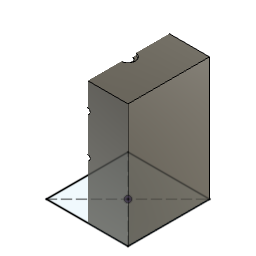
Ikea Stubby Leg v1 (Autodesk Fusion 360 design; units mm, degrees)
Autodesk Fusion 360 part; units mm, degrees
sketch "Sketch1" plane through (0, 0, 0) normal (0, 0, 1) x (1, 0, 0)
  line L0 (25.2, -25.2) -> (-25.2, -25.2)
  line L1 (-25.2, -25.2) -> (-25.2, 25.2)
  line L2 (-25.2, 25.2) -> (25.2, 25.2)
  line L3 (25.2, 25.2) -> (25.2, -25.2)
  line L4 (25.2, -25.2) -> (-25.2, 25.2) construction
  line L5 (-25.2, -25.2) -> (25.2, 25.2) construction
  dimension "d1" = 50.4
  dimension "d2" = 50.4
  constraint horizontal L0
  constraint perpendicular L0 L1
  constraint parallel L0 L2
  constraint parallel L1 L3
  constraint coincident L4 origin
  constraint coincident L5 origin
  measures "d1" distance of L1.end L2.end
  measures "d2" distance of L0.end L1.end
extrude "Extrude1" add sketch "Sketch1" along normal blind 76.2
move_body "Align1" bodies 1 to x (1, 0, 0) y (0, 1, 0) z (0, 0, 1) at (0, 0, 0)
coil "CoilPrimitive1" cut diameter 5.4 section triangle out size 1.5 outside turns 14 pitch 3.2 right hand placed x (1, 0, 0) y (0, 1, 0) z (0, 0, 1) at (0, 0, 0)
cylinder "CylinderPrimitive1" cut diameter 5.4 height 45 placed x (1, 0, 0) y (0, 1, 0) z (0, 0, 1) at (0, 0, 0)
cylinder "CylinderPrimitive2" cut diameter 9 height 1.3 placed x (1, 0, 0) y (0, 1, 0) z (0, 0, 1) at (0, 0, 0)
sketch "Sketch14" plane through (-25.2, 0, 0) normal (-1, 0, 0) x (0, -1, 0)
  line L0 (-25.2, 0) -> (25.2, 0)
  line L1 (25.2, 0) -> (25.2, 76.2)
  line L2 (25.2, 76.2) -> (-25.2, 76.2)
  line L3 (-25.2, 76.2) -> (-25.2, 0)
  point P0 (0, 41.2)
  point P1 (0, 16.2)
  dimension "d21" = 35
  dimension "d22" = 25
  constraint vertical P0 P1
  measures "d21" distance of L2 P0
  measures "d22" distance of P0 P1
sketch "Sketch15" plane through (0, 25.2, 0) normal (0, 1, 0) x (-1, 0, 0)
  line L0 (-25.2, 0) -> (25.2, 0)
  line L1 (25.2, 0) -> (25.2, 76.2)
  line L2 (25.2, 76.2) -> (-25.2, 76.2)
  line L3 (-25.2, 76.2) -> (-25.2, 0)
  point P0 (0, 41.2)
  point P1 (0, 16.2)
  dimension "d23" = 35
  dimension "d24" = 25
  constraint vertical P0 P1
  measures "d23" distance of L2 P0
  measures "d24" distance of P0 P1
hole "Hole3" at (0, 25.2, 41.2) at (0, 25.2, 16.2) direction (0, -1, 0) diameter 3.45 depth 19 tip angle 118
hole "Hole4" at (-25.2, 0, 41.2) at (-25.2, 0, 16.2) direction (1, 0, 0) diameter 3.45 depth 19 tip angle 118
move_body "Align2" bodies 1 to x (1, 0, 0) y (0, -1, 0) z (0, 0, -1) at (0, 0, 76.2)
equation "holedepth = 19 mm"
equation "d26 = holedepth"
named bodies: "Prusa Stand"
